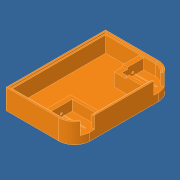
# Autodesk Inventor part: P1794_001
Saved by Autodesk Inventor 2019 (Build 230136000, 136)
## iProperties
Created: 2019-04-29
Part Number: P1794_001
Material: PLA
Document SubType Name: Modeling
Designer: Joan.MAILLARD
Density: 1.25 g/cm^3
Appearance: Orange
Project: P1704 Manette
Description: Bas manette
Author: Joan.MAILLARD
Title: P1704_001_basManette
Autodesk Inventor part; units mm, degrees
ref_plane "YZ Plane" through (0, 0, 0) normal (1, 0, 0) x (0, 1, 0)
ref_plane "XZ Plane" through (0, 0, 0) normal (0, 1, 0) x (-1, 0, 0)
ref_plane "XY Plane" through (0, 0, 0) normal (0, 0, 1) x (1, 0, 0)
sketch "Esquisse1" plane through (0, 0, 0) normal (0, 1, 0) x (-1, 0, 0)
  line L0 (55, 80) -> (55, -80)
  line L1 (-55, -80) -> (-55, 80)
  line L2 (-55, 80) -> (55, -80) construction
  line L3 (55, 80) -> (-55, -80) construction
  line L4 (0, 0) -> (-55, 0) construction
  arc A0 (-55, -55) -> (-30, -80) centre (-30, -55) ccw
  line L5 (-30, -80) -> (55, -80)
  line L6 (-30, -80) -> (-30, -55) construction
  line L7 (55, 80) -> (-30, 80)
  arc A1 (-30, 80) -> (-55, 55) centre (-30, 55) ccw
  line L8 (-30, 55) -> (-30, 80) construction
  dimension "d0" = 160
  dimension "d1" = 110
  dimension "d126" = 25
  dimension "d127" = 25
  constraints: 18 end point, 4 point on circle, 3 horizontal, 3 midpoint, 2 centre point, 2 parallel, 2 point on line, 2 tangent, 2 vertical, 1 perpendicular
  measures "d0" distance of L0.start L0.end
  measures "d1" distance of L0.end L1.start
  measures "d126" distance of L5.start L6.end
  measures "d127" distance of L8.start L7.end
extrude "Extrusion1" add sketch "Esquisse1" along normal blind 32.5
sketch "Esquisse2" plane through (0, 32.5, 0) normal (0, 1, 0) x (1, 0, 0)
  line L0 (-50, 75) -> (-50, -75)
  line L1 (-55, 80) -> (-55, -80) projected
  line L2 (30, 80) -> (-55, 80) projected
  line L3 (-50, -75) -> (30, -75)
  line L4 (30, -75) -> (30, -80) construction
  line L5 (-55, -80) -> (30, -80) construction
  line L6 (-50, 75) -> (30, 75)
  line L7 (30, 75) -> (30, 80) construction
  arc A0 (50, 55) -> (30, 75) centre (30, 55) ccw
  line L8 (30, 75) -> (30, 55) construction
  arc A1 (55, 55) -> (30, 80) centre (30, 55) ccw construction
  line L9 (50, 55) -> (50, -55)
  line L10 (55, 55) -> (50, 55) construction
  line L11 (50, -55) -> (55, -55) construction
  arc A2 (30, -75) -> (50, -55) centre (30, -55) ccw
  line L12 (55, -55) -> (55, 55) construction
  point P0 (0, 0)
  dimension "d67" = 5
  dimension "d131" = 5
  constraints: 18 end point, 4 horizontal, 4 point on circle, 3 vertical, 2 centre point, 2 tangent, 1 coincident, 1 concentric, 1 parallel, 1 perpendicular
  measures "d67" distance between parallel lines of L1 L0
  measures "d131" distance between parallel lines of L12 L9
extrude "Extrusion2" cut sketch "Esquisse2" against normal blind 27.5
sketch "Esquisse6" plane through (0, 5, 0) normal (0, 1, 0) x (1, 0, 0)
  line L0 (50, 40) -> (11.25, 40)
  line L1 (11.25, 40) -> (11.25, 35)
  line L2 (11.25, 35) -> (50, 35)
  line L3 (50, 35) -> (50, 40)
  line L4 (11.25, 35) -> (3.75, 35)
  line L5 (3.75, 35) -> (3.75, 75)
  line L6 (3.75, 75) -> (11.25, 75)
  line L7 (11.25, 75) -> (11.25, 35)
  line L8 (11.25, -75) -> (3.75, -75)
  line L9 (3.75, -75) -> (3.75, -35)
  line L10 (3.75, -35) -> (11.25, -35)
  line L11 (11.25, -35) -> (11.25, -75)
  line L12 (50, -35) -> (11.25, -35)
  line L13 (11.25, -35) -> (11.25, -40)
  line L14 (11.25, -40) -> (50, -40)
  line L15 (50, -40) -> (50, -35)
  line L16 (11.25, -75) -> (80.7095, -75) construction
  line L17 (50, -40) -> (50, -93.5027) construction
  line L18 (30, -75) -> (-50, -75) construction
  line L19 (50, 55) -> (50, -55) construction
  line L20 (-50, 75) -> (30, 75) construction
  point P0 (0, 0)
  point P1 (7.5, -35)
  dimension "d44" = 5
  dimension "d45" = 7.5
  dimension "d48" = 5
  dimension "d50" = 7.5
  dimension "d132" = 35
  dimension "d133" = 38.75
  dimension "d134" = 38.75
  dimension "d135" = 35
  constraints: 36 end point, 8 parallel, 5 horizontal, 5 point on line, 4 perpendicular, 1 midpoint, 1 vertical
  measures "d44" distance between parallel lines of L2 L0
  measures "d45" distance between parallel lines of L5 L7
  measures "d48" distance between parallel lines of L14 L12
  measures "d50" distance between parallel lines of L11 L9
  measures "d132" distance between parallel lines of L14 L16
  measures "d133" distance between parallel lines of L11 L17
  measures "d134" distance of L0.start L0.end
  measures "d135" distance between parallel lines of L20 L0
extrude "Extrusion4" add sketch "Esquisse6" along normal blind 24
sketch "Esquisse11" plane through (55, 0, 55) normal (1, 0, 0) x (0, 0, -1)
  line L0 (-12.5, 32.5) -> (7.5, 32.5)
  line L1 (7.5, 32.5) -> (7.5, 12.5)
  line L2 (7.5, 12.5) -> (-12.5, 12.5)
  line L3 (-12.5, 12.5) -> (-12.5, 32.5)
  line L4 (122.5, 32.5) -> (102.5, 32.5)
  line L5 (102.5, 32.5) -> (102.5, 12.5)
  line L6 (102.5, 12.5) -> (122.5, 12.5)
  line L7 (122.5, 12.5) -> (122.5, 32.5)
  line L8 (0, 0) -> (110, 0) projected
  line L9 (0, 32.5) -> (110, 32.5) projected
  line L10 (135, 0) -> (110, 0) projected
  line L11 (135, 32.5) -> (110, 32.5) projected
  line L12 (-25, 0) -> (-25, 32.5) projected
  line L13 (135, 0) -> (135, 32.5) projected
  line L14 (71.6904, 12.5) -> (52.7334, 12.5) construction
  dimension "d138" = 20
  dimension "d139" = 20
  dimension "d140" = 12.5
  dimension "d141" = 12.5
  dimension "d154" = 12.5
  constraints: 18 end point, 4 parallel, 3 collinear, 3 horizontal, 2 perpendicular, 1 coincident, 1 midpoint, 1 point on line
  measures "d138" distance between parallel lines of L3 L1
  measures "d139" distance between parallel lines of L7 L5
  measures "d140" distance between parallel lines of L12 L3
  measures "d141" distance between parallel lines of L13 L7
  measures "d154" distance between parallel lines of L14 L10
extrude "Extrusion6" cut sketch "Esquisse11" against normal blind 20
sketch "Esquisse16" plane through (11.25, 5, 75) normal (1, 0, 0) x (0, 0, -1)
  line L0 (17.5, 12.5) -> (7.5, 12.5) construction
  line L1 (17.5, 12.5) -> (27.5, 12.5) construction
  line L2 (130, 0) -> (122.5, 0) construction
  line L3 (7.5, 7.5) -> (7.5, 27.5) projected
  line L4 (27.5, 27.5) -> (27.5, 7.5) projected
  line L5 (7.5, 6) -> (20, 6) projected
  line L6 (27.5, 7.5) -> (20, 7.5) projected
  point P0 (75, -5)
  point P1 (130, 6)
  point P2 (122.5, 6)
  point P3 (27.5, 6)
  point P4 (27.5, -5)
  dimension "d174" = 5
  constraints: 4 end point, 3 point on line, 1 collinear, 1 horizontal, 1 other
  measures "d174" distance between parallel lines of L1 L6
hole "Perçage6" at (11.25, 17.5, 57.5) direction (-1, 0, 0) diameter 3.4 depth 10
sketch "Esquisse17" plane through (11.25, 5, -40) normal (1, 0, 0) x (0, 0, -1)
  line L0 (27.5, 27.5) -> (27.5, 7.5) projected
  line L1 (7.5, 7.5) -> (7.5, 27.5) projected
  line L2 (5.8848, 12.5) -> (-4.3187, 12.5) construction
  line L3 (15, 7.5) -> (15, 7.5) projected
  line L4 (17.5, 12.5) -> (7.5, 12.5) construction
  line L5 (17.5, 12.5) -> (27.5, 12.5) construction
  point P0 (-40, -5)
  point P1 (7.5, 6)
  point P2 (-87.5, 6)
  point P3 (27.5, -5)
  point P4 (7.5, -5)
  dimension "d155" = 5
  constraints: 6 end point, 3 point on line, 2 perpendicular, 1 collinear, 1 horizontal, 1 horizontal alignment
hole "Perçage7" at (11.25, 17.5, -57.5) direction (-1, 0, 0) diameter 3.4 depth 10
sketch "Esquisse20" plane through (0, 32.5, 0) normal (0, 1, 0) x (1, 0, 0)
  line L0 (-52.5, 77.5) -> (-52.5, -77.5)
  line L1 (-52.5, -77.5) -> (30, -77.5)
  arc A0 (30, -77.5) -> (52.5, -55) centre (30, -55) ccw
  line L2 (52.5, -55) -> (52.5, 55)
  arc A1 (52.5, 55) -> (30, 77.5) centre (30, 55) ccw
  line L3 (-52.5, 77.5) -> (30, 77.5)
  line L4 (30, 80) -> (30, 75) construction
  arc A2 (45.6125, 67.5) -> (30, 75) centre (30, 55) ccw construction
  line L5 (30, -80) -> (30, -75) construction
  arc A3 (30, -80) -> (51.6506, -67.5) centre (30, -55) ccw construction
  arc A4 (51.6506, 67.5) -> (30, 80) centre (30, 55) ccw construction
  line L6 (-50, 0) -> (-55, 0) construction
  line L7 (-55, 0) -> (-50, 0) construction
  line L8 (-50, -75) -> (-50, 75) construction
  line L9 (-55, 80) -> (-55, -80) construction
  line L10 (30, 75) -> (-50, 75)
  line L11 (-50, -75) -> (30, -75)
  arc A5 (50, 55) -> (30, 75) centre (30, 55) ccw
  arc A6 (30, -75) -> (50, -55) centre (30, -55) ccw
  line L12 (50, -55) -> (50, 55)
  point P0 (0, 0)
  point P1 (-52.5, 0)
  constraints: 22 end point, 12 point on circle, 6 midpoint, 5 horizontal, 5 tangent, 4 centre point, 4 vertical, 3 concentric, 2 coincident, 2 equal radius, 2 parallel, 1 collinear
extrude "Extrusion12" cut sketch "Esquisse20" against normal blind 2
sketch "Esquisse22" plane through (0, 5, 0) normal (0, 1, 0) x (1, 0, 0)
  line L0 (11.25, -75) -> (11.25, -40) projected
  line L1 (11.25, -40) -> (11.25, -75) projected
  line L2 (30, -75) -> (11.25, -75) projected
  arc A0 (30, -75) -> (50, -55) centre (30, -55) ccw projected
  line L3 (50, -40) -> (50, -55) projected
  line L4 (50, -40) -> (11.25, -40) projected
  line L5 (11.25, 75) -> (11.25, 40) projected
  line L6 (11.25, 40) -> (50, 40) projected
  line L7 (50, 55) -> (50, 40) projected
  arc A1 (50, 55) -> (30, 75) centre (30, 55) ccw projected
  line L8 (11.25, 75) -> (30, 75) projected
  point P0 (0, 0)
extrude "Extrusion14" add sketch "Esquisse22" along normal blind 7.5
sketch "Esquisse24" plane through (55, 12.5, 55) normal (0, 1, 0) x (1, 0, 0)
  line L0 (-9.3875, -7.5596) -> (-9.3875, 12.2233) construction
  line L1 (-43.75, -7.1) -> (-9.3875, -7.1)
  line L2 (-9.3875, -7.1) -> (-9.3875, -6.1)
  line L3 (-9.3875, -6.1) -> (-43.75, -6.1)
  line L4 (-43.75, -6.1) -> (-43.75, -7.1)
  line L5 (-43.75, 1.1) -> (-9.3875, 1.1)
  line L6 (-9.3875, 1.1) -> (-9.3875, 2.1)
  line L7 (-9.3875, 2.1) -> (-43.75, 2.1)
  line L8 (-43.75, 2.1) -> (-43.75, 1.1)
  line L9 (-43.75, -20) -> (-43.75, 15) construction
  line L10 (-43.75, 15) -> (-5, 15) projected
  line L11 (-43.75, 107.9) -> (-9.3875, 107.9)
  line L12 (-9.3875, 107.9) -> (-9.3875, 108.9)
  line L13 (-9.3875, 108.9) -> (-43.75, 108.9)
  line L14 (-43.75, 108.9) -> (-43.75, 107.9)
  line L15 (-43.75, 116.1) -> (-9.3875, 116.1)
  line L16 (-9.3875, 116.1) -> (-9.3875, 117.1)
  line L17 (-9.3875, 117.1) -> (-43.75, 117.1)
  line L18 (-43.75, 117.1) -> (-43.75, 116.1)
  line L19 (-5, 95) -> (-43.75, 95) projected
  line L20 (-43.75, 95) -> (-43.75, 130) projected
  point P0 (-9.3875, -12.5)
  point P1 (-43.75, 1.6)
  point P2 (-43.75, -6.6)
  point P3 (-9.3875, 1.6)
  point P4 (-9.3875, -6.6)
  point P5 (-9.3875, 108.4)
  point P6 (-9.3875, 116.6)
  point P7 (-43.75, 108.4)
  dimension "d160" = 1
  dimension "d161" = 1
  dimension "d162" = 7.2
  dimension "d163" = 12.9
  dimension "d164" = 1
  dimension "d165" = 1
  dimension "d166" = 7.2
  dimension "d167" = 12.9
  constraints: 34 end point, 9 point on line, 8 parallel, 7 midpoint, 4 horizontal, 4 perpendicular, 1 vertical
  measures "d160" distance of L1.end L2.end
  measures "d161" distance of L5.end L6.end
  measures "d162" distance between parallel lines of L3 L5
  measures "d163" distance between parallel lines of L10 L7
  measures "d164" distance of L15.end L16.end
  measures "d165" distance of L11.end L12.end
  measures "d166" distance between parallel lines of L15 L13
  measures "d167" distance between parallel lines of L11 L19
extrude "Extrusion15" add sketch "Esquisse24" along normal blind 0.9
sketch "Esquisse25" plane through (0, 29, 0) normal (0, 1, 0) x (1, 0, 0)
  line L0 (3.75, 35) -> (23.25, 35)
  line L1 (23.25, 35) -> (23.25, 49)
  line L2 (23.25, 49) -> (3.75, 49)
  line L3 (3.75, 49) -> (3.75, 35)
  line L4 (3.75, 75) -> (3.75, 35) construction
  line L5 (3.75, 35) -> (50, 35) construction
  point P0 (0, 0)
  dimension "d170" = 14
  dimension "d171" = 19.5
  constraints: 8 end point, 2 collinear, 2 parallel, 1 horizontal, 1 perpendicular
  measures "d170" distance of L0.end L1.end
  measures "d171" distance between parallel lines of L3 L1
extrude "Extrusion16" cut sketch "Esquisse25" against normal blind 3
equation "\"d67\" = d66"
equation "\"d131\" = d67"
equation "\"d45\" = 1.5 * d44"
equation "\"d48\" = d44"
equation "\"d50\" = d45"
equation "\"d134\" = d133"
equation "\"d135\" = d132"
equation "\"d139\" = d138"
equation "\"d141\" = d140"
equation "\"d66\" = 5"
